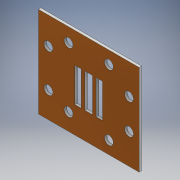
# Autodesk Inventor part: valvle plate
Saved by Autodesk Inventor 2017 (Build 210142000, 142)
## iProperties
Created: 2018-11-06
Part Number: valvle plate
Material: Generic
Document SubType Name: Modeling
Designer: User
Density: 1 g/cm^3
Appearance: Default
Author: User
Autodesk Inventor part; units mm, degrees
ref_plane "YZ Plane" through (0, 0, 0) normal (1, 0, 0) x (0, 1, 0)
ref_plane "XZ Plane" through (0, 0, 0) normal (0, 1, 0) x (-1, 0, 0)
ref_plane "XY Plane" through (0, 0, 0) normal (0, 0, 1) x (1, 0, 0)
sketch "Sketch1" plane through (0, 0, 0) normal (0, 1, 0) x (-1, 0, 0)
  line L0 (0, 0) -> (0, -36)
  line L1 (0, -36) -> (-40, -36)
  line L2 (-40, -36) -> (-40, 0)
  line L3 (-40, 0) -> (0, 0)
  line L4 (0, -18) -> (-40, -18) construction
  line L5 (-20, 0) -> (-20, -36) construction
  circle A0 centre (-36, -12) radius 1.75
  circle A1 centre (-36, -24) radius 1.75
  circle A2 centre (-4, -10.7051) radius 1.75
  circle A3 centre (-4, -25.75) radius 1.75
  circle A4 centre (-28, -5) radius 1.75
  circle A5 centre (-12, -5.4968) radius 1.75
  circle A6 centre (-28, -31) radius 1.75
  circle A7 centre (-12, -29.25) radius 1.75
  line L6 (-20, -18) -> (-18.5, -18) construction
  line L7 (-20, -18) -> (-21.5, -18) construction
  line L8 (-18.5, -12) -> (-18.5, -25.5) construction
  line L9 (-18.5, -12) -> (-18.5, -25.5)
  line L10 (-18.5, -25.5) -> (-21.5, -25.5)
  line L11 (-21.5, -25.5) -> (-21.5, -12)
  line L12 (-21.5, -12) -> (-18.5, -12)
  line L13 (-18.5, -16.9522) -> (-17, -16.9522) construction
  line L14 (-21.5, -16.9522) -> (-23, -16.9522) construction
  line L15 (-23, -12) -> (-23, -25.5) construction
  line L16 (-23, -12) -> (-23, -25.5)
  line L17 (-23, -25.5) -> (-25.5, -25.5)
  line L18 (-25.5, -25.5) -> (-25.5, -12)
  line L19 (-25.5, -12) -> (-23, -12)
  line L20 (-17, -12) -> (-17, -25.5)
  line L21 (-17, -25.5) -> (-14.5, -25.5)
  line L22 (-14.5, -25.5) -> (-14.5, -12)
  line L23 (-14.5, -12) -> (-17, -12)
  dimension "d0" = 36
  dimension "d1" = 40
  dimension "d4" = 3.5
  dimension "d5" = 6
  dimension "d7" = 3.5
  dimension "d8" = 3.5
  dimension "d14" = 32
  dimension "d15" = 4
  dimension "d16" = 4
  dimension "d17" = 4
  dimension "d19" = 3.5
  dimension "d20" = 3.5
  dimension "d21" = 3.5
  dimension "d23" = 5
  dimension "d24" = 5
  dimension "d28" = 16
  dimension "d29" = 12
  dimension "d30" = 3.5
  dimension "d31" = 16
  dimension "d32" = 10.7051
  dimension "d33" = 25.75
  dimension "d34" = 5.4968
  dimension "d35" = 29.25
  dimension "d42" = 3
  dimension "d45" = 1.5
  dimension "d53" = 2.5
  dimension "d54" = 90
  dimension "d56" = 23
  dimension "d61" = 12
  dimension "d62" = 12
  dimension "d66" = 13.5
  dimension "d67" = 2.5
  dimension "d70" = 14.5
  dimension "d71" = 4.9522
  dimension "d72" = 24
  dimension "d73" = 13.5
  dimension "d74" = 4.9522
  dimension "d75" = 0
  dimension "d76" = 13.5
  dimension "d77" = 17
  dimension "d78" = 18.5
  dimension "d79" = 21.5
  dimension "d80" = 23
  dimension "d81" = 12
  constraints: 48 end point, 14 perpendicular, 8 centre point, 5 midpoint, 4 point on line, 3 vertical, 2 collinear, 1 equal radius
  measures "d0" distance of L0.start L0.end
  measures "d1" distance of L0.end L1.end
  measures "d4" diameter of A1
  measures "d5" distance from line of L4 A0.centre
  measures "d7" diameter of A2
  measures "d8" diameter of A3
  measures "d14" horizontal distance of A2.centre A0.centre
  measures "d15" distance from line of L0 A2.centre
  measures "d16" distance from line of L2 A1.centre
  measures "d17" distance from line of L0 A3.centre
  measures "d19" diameter of A4
  measures "d20" diameter of A5
  measures "d21" diameter of A6
  measures "d23" distance from line of L1 A6.centre
  measures "d24" distance from line of L3 A4.centre
  measures "d28" horizontal distance of A5.centre A4.centre
  measures "d29" distance from line of L0 A5.centre
  measures "d30" diameter of A7
  measures "d31" horizontal distance of A6.centre A7.centre
  measures "d32" distance from line of A2.centre L3
  measures "d33" distance from line of A3.centre L3
  measures "d34" distance from line of A5.centre L3
  measures "d35" distance from line of A7.centre L3
  measures "d42" distance of L8.end L10.end
  measures "d45" distance from line of L9 L6.start
  measures "d53" distance of L15.end L17.end
  measures "d54" angle of L12 L0
  measures "d56" distance between parallel lines of L16 L0
  measures "d61" distance from line of L0.start L12
  measures "d62" distance from line of A7.centre L0
  measures "d66" distance of L20.start L20.end
  measures "d67" distance of L20.end L21.end
  measures "d70" distance between parallel lines of L22 L0
  measures "d71" distance between parallel lines of L13 L23
  measures "d72" distance between parallel lines of L23 L1
  measures "d73" distance between parallel lines of L23 L10
  measures "d74" distance between parallel lines of L14 L23
  measures "d75" distance between parallel lines of L23 L19
  measures "d76" distance between parallel lines of L23 L17
  measures "d77" distance from line of L13.end L0
  measures "d78" distance from line of L6.end L0
  measures "d79" distance from line of L7.end L0
  measures "d80" distance from line of L14.end L0
  measures "d81" distance from line of A1.centre L23
extrude "Extrusion3" add sketch "Sketch1" along normal blind 1
body "Solid3"
